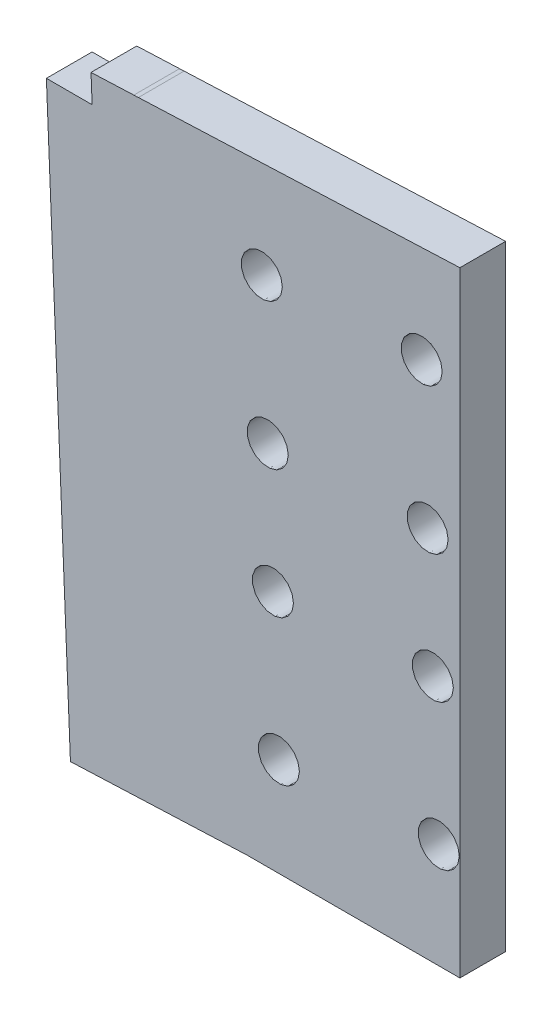
# Autodesk Inventor part: cable_mount
Saved by Autodesk Inventor 2019 (Build 230136000, 136)
## iProperties
Created: 2020-04-25
Part Number: cable_mount
Material: Generisch
Document SubType Name: Modeling
Designer: marc
Density: 1 g/cm^3
Appearance: Vorgabe
Author: marc
Autodesk Inventor part; units mm, degrees
ref_plane "YZ Plane" through (0, 0, 0) normal (1, 0, 0) x (0, 1, 0)
ref_plane "XZ Plane" through (0, 0, 0) normal (0, 1, 0) x (-1, 0, 0)
ref_plane "XY Plane" through (0, 0, 0) normal (0, 0, 1) x (1, 0, 0)
sketch "Skizze1" plane through (0, 0, 0) normal (0, 0, 1) x (1, 0, 0)
  ellipse E0 centre (-12.1961, -42.2319) end of major axis (-9.6527, -42.1265) minor radius 1.8 (-13.7003, -43.7155) -> (-13.818, -40.878) ccw projected
  arc A0 (-13.818, -40.878) -> (-13.7003, -43.7155) centre (-14.8644, -42.3426) ccw projected
  ellipse E1 centre (-12.6519, -31.2414) end of major axis (-10.1085, -31.1359) minor radius 1.8 (-14.1561, -32.725) -> (-14.2737, -29.8874) ccw projected
  arc A1 (-14.2737, -29.8874) -> (-14.1561, -32.725) centre (-15.3201, -31.352) ccw projected
  ellipse E2 centre (-13.1697, -18.7521) end of major axis (-10.6263, -18.6467) minor radius 1.8 (-14.6739, -20.2357) -> (-14.7916, -17.3982) ccw projected
  arc A2 (-14.7916, -17.3982) -> (-14.6739, -20.2357) centre (-15.838, -18.8628) ccw projected
  ellipse E3 centre (-11.6782, -54.7212) end of major axis (-9.1348, -54.6157) minor radius 1.8 (-13.1824, -56.2048) -> (-13.3001, -53.3673) ccw projected
  arc A3 (-13.3001, -53.3673) -> (-13.1824, -56.2048) centre (-14.3465, -54.8319) ccw projected
  line L0 (1.4946, -9.6367) -> (3.6905, -62.5912) projected
  line L1 (1.4946, -9.6367) -> (-19.2875, -10.4985) projected
  line L2 (-19.2875, -10.4985) -> (-17.0916, -63.453) projected
  line L3 (-17.0916, -63.453) -> (3.6905, -62.5912) projected
  circle A4 centre (-0.8764, -41.7626) radius 1.8 projected
  circle A5 centre (-1.3321, -30.772) radius 1.8 projected
  circle A6 centre (-1.85, -18.2827) radius 1.8 projected
  circle A7 centre (-0.3585, -54.2518) radius 1.8 projected
  line L4 (1.4946, -9.6367) -> (-17.0916, -9.6367)
  line L5 (-17.0916, -9.6367) -> (-17.0916, -63.453)
  line L6 (-17.0916, -63.453) -> (1.4946, -63.453)
  line L7 (1.4946, -63.453) -> (1.4946, -9.6367)
  circle A8 centre (-0.3585, -54.2518) radius 1.8
  circle A9 centre (-0.8764, -41.7626) radius 1.8
  circle A10 centre (-1.3321, -30.772) radius 1.8
  circle A11 centre (-1.85, -18.2827) radius 1.8
  circle A12 centre (-15.838, -18.8628) radius 1.8
  circle A13 centre (-15.3201, -31.352) radius 1.8
  circle A14 centre (-14.8644, -42.3426) radius 1.8
  circle A15 centre (-14.3465, -54.8319) radius 1.8
  point P0 (0, 0)
  constraints: 8 centre point, 8 coincident, 8 concentric, 8 end point, 2 parallel, 1 horizontal, 1 perpendicular, 4 other
extrude "Extrusion1" add sketch "Skizze1" along normal blind 4 contours A14 E0 | A13 E1 | E1 A1 L5 A2 E2 L1 L7 L3 | L5 L2 L1 A2 A1 | L3 L7 L6 | A12 E2 | A15 E3
sketch "Skizze2" plane through (1.4946, -9.6367, 0) normal (1, 0, 0) x (0, 0, 1)
  line L0 (0, 0.8618) -> (0, 53.8163) projected
  line L1 (0, 0.8618) -> (19, 0.8618)
  line L2 (19, 0.8618) -> (19, 53.8163)
  line L3 (19, 53.8163) -> (0, 53.8163)
  line L4 (0, 53.8163) -> (0, 0.8618)
  line L5 (4, 53.8163) -> (4, 0) projected
  point P0 (0, -9.6367)
  dimension "d3" = 15
  constraints: 6 end point, 1 horizontal, 1 parallel, 1 point on line, 1 vertical, 3 other
  measures "d3" distance between parallel lines of L2 L5
extrude "Extrusion2" [suppressed]
sketch "Skizze3" plane through (-6.3, -26.5, 0) normal (1, 0, 0) x (0, 0, -1)
  line L0 (-7, 52) -> (-15, 52)
  line L1 (-15, 52) -> (-15, 35)
  line L2 (-15, 35) -> (-7, 35)
  line L3 (-7, 35) -> (-7, 52)
  line L4 (-4, 53) -> (-4, 0) projected
  line L5 (-19, 53) -> (-4, 53) projected
  circle A0 centre (-11, 31) radius 1.5
  point P0 (0, 26.5)
  dimension "d6" = 8
  dimension "d7" = 17
  dimension "d8" = 3
  dimension "d9" = 1
  dimension "d10" = 4
  dimension "d11" = 3
  dimension "d12" = 4
  constraints: 8 end point, 2 parallel, 1 centre point, 1 horizontal, 1 perpendicular
  measures "d6" distance of L2.end L1.end
  measures "d7" distance of L1.end L0.end
  measures "d8" distance between parallel lines of L4 L3
  measures "d9" distance between parallel lines of L5 L0
  measures "d10" distance from line of L2 A0.centre
  measures "d11" diameter of A0
  measures "d12" distance from line of L3 A0.centre
extrude "Extrusion3" [suppressed]
ref_plane "Arbeitsebene1" through (-1296.3098, -63.453, 4) normal (0.0207202, -0.9997853, 0) x (0, 0, 1)
mirror "Spiegeln1" [suppressed]
sketch "Skizze4" plane through (-19.2875, -10.4985, 0) normal (-0.9991413, -0.0414316, 0) x (0, 0, -1)
  line L0 (0, 0) -> (0, 53) projected
  line L1 (0, 53) -> (-4, 53) projected
  line L2 (-4, 0) -> (-4, 53) projected
  line L3 (0, 0) -> (-4, 0) projected
  point P0 (0, -9.6904)
extrude "Extrusion4" add sketch "Skizze4" along normal blind 15.5
sketch "Skizze5" plane through (0, 0, 4) normal (0, 0, 1) x (1, 0, 0)
  line L0 (-30.6781, -13.3745) -> (-38.5781, -13.3745)
  line L1 (-38.5781, -13.3745) -> (-39.6071, 11.4403)
  line L2 (-39.6071, 11.4403) -> (-31.7139, 11.6041)
  line L3 (-31.7139, 11.6041) -> (-30.6781, -13.3745)
  line L4 (-32.5783, -64.0952) -> (-34.7742, -11.1407) projected
  line L5 (-17.0916, -63.453) -> (-32.5783, -63.453) projected
  line L6 (1.4946, -9.6367) -> (-34.7742, -11.1407) projected
  circle A0 centre (-26.901, -9.1245) radius 1.7
  circle A1 centre (-28.2889, 24.3468) radius 1.7
  point P0 (0, 0)
  point P1 (-6.3, 26.5)
  point P2 (-6.3, -26.5)
  point P3 (1.4946, -9.6367)
  dimension "d26" = 7.9
  dimension "d27" = 25
  dimension "d28" = 14
  dimension "d29" = 53
  dimension "d30" = 3.95
  dimension "d31" = 3.95
  dimension "d32" = 33.5
  dimension "d33" = 3.4
  dimension "d34" = 3.4
  dimension "d35" = 4.25
  dimension "d41" = 4
  constraints: 8 end point, 2 centre point, 1 horizontal, 1 parallel, 4 other
  measures "d26" distance of L0.start L0.end
  measures "d27" distance of L2.end L0.start
  measures "d29" distance of L4.start L4.end
  measures "d30" distance from line of L3 A1.centre
  measures "d31" distance from line of L3 A0.centre
  measures "d32" distance of A1.centre A0.centre
  measures "d33" diameter of A0
  measures "d34" diameter of A1
  measures "d35" distance from line of L0 A0.centre
  measures "d41" distance between parallel lines of L4 L3
extrude "Extrusion5" cut sketch "Skizze5" against normal blind 4
equation "\"d12\" = 0.5 * d6"
equation "\"d28\" = -0.5 * d27 + 0.5 * d29"
equation "\"d30\" = 0.5 * d26"
equation "\"d31\" = d30"
equation "\"d34\" = d33"
equation "\"d35\" = 0.5 * d32 - 0.5 * d27"
